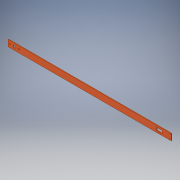
# Autodesk Inventor part: convyerwall2
Saved by Autodesk Inventor 2019 (Build 230136000, 136)
## iProperties
Created: 2021-11-02
Part Number: convyerwall2
Material: Generic
Document SubType Name: Modeling
Designer: modym
Density: 1 g/cm^3
Appearance: Smooth - Light Orange
Author: modym
Autodesk Inventor part; units mm, degrees
ref_plane "YZ Plane" through (0, 0, 0) normal (1, 0, 0) x (0, 1, 0)
ref_plane "XZ Plane" through (0, 0, 0) normal (0, 1, 0) x (-1, 0, 0)
ref_plane "XY Plane" through (0, 0, 0) normal (0, 0, 1) x (1, 0, 0)
sketch "Sketch1" plane through (0, 0, 0) normal (0, 0, 1) x (1, 0, 0)
  line L0 (0, 0) -> (1300, 0)
  line L1 (1300, 0) -> (1300, 50)
  line L2 (1300, 50) -> (0, 50)
  line L3 (0, 50) -> (0, 0)
  circle A0 centre (50, 25) radius 10.5
  circle A1 centre (1288, 40) radius 3
  circle A2 centre (1288, 10) radius 3
  line L4 (1182.5, 14.5) -> (1227.5, 14.5)
  line L5 (1227.5, 14.5) -> (1227.5, 35.5)
  line L6 (1227.5, 35.5) -> (1182.5, 35.5)
  line L7 (1182.5, 35.5) -> (1182.5, 14.5)
  circle A3 centre (14.5, 25) radius 5
  circle A4 centre (85.5, 25) radius 5
  dimension "d0" = 1300
  dimension "d1" = 50
  dimension "d2" = 21
  dimension "d3" = 6
  dimension "d4" = 6
  dimension "d5" = 45
  dimension "d6" = 21
  dimension "d7" = 14.5
  dimension "d8" = 72.5
  dimension "d13" = 10
  dimension "d14" = 10
  constraints: 16 end point, 5 centre point, 4 parallel, 2 horizontal, 2 perpendicular
  measures "d0" distance of L2.end L1.end
  measures "d1" distance of L1.end L0.end
  measures "d2" diameter of A0
  measures "d3" diameter of A1
  measures "d4" diameter of A2
  measures "d5" distance of L6.end L5.end
  measures "d6" distance of L5.end L4.end
  measures "d7" distance between parallel lines of L0 L4
  measures "d8" distance between parallel lines of L1 L5
  measures "d13" diameter of A3
  measures "d14" diameter of A4
extrude "Extrusion2" add sketch "Sketch1" along normal blind 5
equation "\"d7\" = -0.5 * d6 + 0.5 * d1"
body "Solid2"
